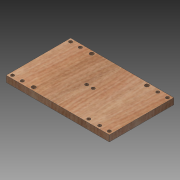
# Autodesk Inventor part: wasteboard
Saved by Autodesk Inventor 2014 (Build 180170000, 170)
## iProperties
Created: 2013-07-14
Part Number: wasteboard
Material: Wood
Document SubType Name: Modeling
Designer: Edward
Density: 0.570257 g/cm^3
Appearance: Birch - Natural Polished
Author: Edward
Autodesk Inventor part; units mm, degrees
ref_plane "YZ Plane" through (0, 0, 0) normal (1, 0, 0) x (0, 1, 0)
ref_plane "XZ Plane" through (0, 0, 0) normal (0, 1, 0) x (-1, 0, 0)
ref_plane "XY Plane" through (0, 0, 0) normal (0, 0, 1) x (1, 0, 0)
sketch "Sketch1" plane through (0, 0, 0) normal (0, 0, 1) x (1, 0, 0)
  line L0 (-160, 100) -> (160, 100)
  line L1 (160, 100) -> (160, -100)
  line L2 (160, -100) -> (-160, -100)
  line L3 (-160, -100) -> (-160, 100)
  point P0 (0, 0)
  dimension "d0" = 320
  dimension "d1" = 200
  dimension "d2" = 160
  dimension "d3" = 100
  constraints: 8 end point, 2 parallel, 1 horizontal, 1 perpendicular
  measures "d0" distance of L1.end L2.end
  measures "d1" distance of L0.end L1.end
  measures "d2" distance from line of L3 point (0, 0)
  measures "d3" distance from line of L0 point (0, 0)
extrude "Extrusion1" add sketch "Sketch1" along normal blind 19.05
sketch "Sketch2" plane through (0, 0, 0) normal (0, 0, -1) x (-1, 0, 0)
  circle A0 centre (150, 90) radius 2.5 projected
  circle A1 centre (85.4, 90.7874) radius 2.0701 projected
  circle A2 centre (85.4, -89.2126) radius 2.5 projected
  circle A3 centre (150, -90) radius 2.5 projected
  circle A4 centre (10, 0) radius 2.067 projected
  circle A5 centre (-10, 0) radius 2.067 projected
  circle A6 centre (-85.4, -89.2126) radius 2.0701 projected
  circle A7 centre (-150, -90) radius 2.5 projected
  circle A8 centre (-85.4, 90.7874) radius 2.0701 projected
  circle A9 centre (-150, 90) radius 2.5 projected
  circle A10 centre (-150, -90) radius 5
  circle A11 centre (-85.4, -89.2126) radius 5
  circle A12 centre (-150, 90) radius 5
  circle A13 centre (-85.4, 90.7874) radius 6
  circle A14 centre (-10, 0) radius 5
  circle A15 centre (10, 0) radius 5
  circle A16 centre (85.4, 90.7874) radius 6
  circle A17 centre (150, 90) radius 5
  circle A18 centre (85.4, -89.2126) radius 6
  circle A19 centre (150, -90) radius 5
  point P0 (0, 0)
  dimension "d6" = 10
  dimension "d7" = 10
  dimension "d8" = 10
  dimension "d9" = 12
  dimension "d10" = 10
  dimension "d11" = 10
  dimension "d12" = 12
  dimension "d13" = 10
  dimension "d14" = 12
  dimension "d15" = 10
  constraints: 10 centre point, 10 coincident
  measures "d6" diameter of A10
  measures "d7" diameter of A11
  measures "d8" diameter of A12
  measures "d9" diameter of A13
  measures "d10" diameter of A14
  measures "d11" diameter of A15
  measures "d12" diameter of A16
  measures "d13" diameter of A17
  measures "d14" diameter of A18
  measures "d15" diameter of A19
extrude "Extrusion2" cut sketch "Sketch2" against normal through all contours A0 | A1 | A2 | A3 | A4 | A5 | A6 | A7 | A8 | A9 | A10 | A11 | A12 | A13 | A14 | A15 | A16 | A17 | A18 | A19
sketch "Sketch5" plane through (0, 0, 19.05) normal (0, 0, 1) x (1, 0, 0)
  circle A0 centre (-120, 90) radius 2.75 projected
  circle A1 centre (-120, -90) radius 2.75 projected
  circle A2 centre (120, -90) radius 2.75 projected
  circle A3 centre (120, 90) radius 2.75 projected
  point P0 (0, 0)
hole "Hole1" at (-120, 90, 19.05) at (-120, -90, 19.05) at (120, -90, 19.05) at (120, 90, 19.05) direction (0, 0, -1) diameter 5 end through all counterbore diameter 10 counterbore depth 12
equation "\"d2\" = 0.5 * d0"
equation "\"d3\" = 0.5 * d1"
body "Solid1"
